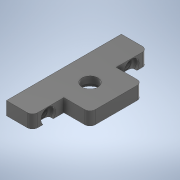
# Autodesk Inventor part: КрепежРадиатора
Saved by Autodesk Inventor 2020 (Build 240168000, 168)
## iProperties
Created: 2020-04-05
Part Number: КрепежРадиатора
Material: Типовые
Document SubType Name: Modeling
Designer: Михаил
Density: 1 g/cm^3
Appearance: По умолчанию
Author: Михаил
Autodesk Inventor part; units mm, degrees
ref_plane "YZ Plane" through (0, 0, 0) normal (1, 0, 0) x (0, 1, 0)
ref_plane "XZ Plane" through (0, 0, 0) normal (0, 1, 0) x (-1, 0, 0)
ref_plane "XY Plane" through (0, 0, 0) normal (0, 0, 1) x (1, 0, 0)
sketch "Эскиз1" plane through (0, 0, 0) normal (0, 1, 0) x (-1, 0, 0)
  line L0 (0, 0) -> (20, 0)
  line L1 (20, 0) -> (20, -20)
  line L2 (20, -20) -> (0, -20)
  line L3 (0, -20) -> (0, 0)
  dimension "d0" = 20
  dimension "d1" = 20
  constraints: 8 end point, 2 parallel, 1 horizontal, 1 perpendicular
  measures "d0" distance of L1.end L2.end
  measures "d1" distance of L0.end L1.end
extrude "Выдавливание1" add sketch "Эскиз1" along normal blind 5
sketch "Эскиз2" plane through (-20, 0, -20) normal (-1, 0, 0) x (0, 0, 1)
  line L0 (0, 5) -> (20, 5) projected
  line L1 (20, 5) -> (32, 5)
  line L2 (32, 5) -> (32, 0)
  line L3 (32, 0) -> (20, 0)
  line L4 (20, 0) -> (20, 5)
  line L5 (0, 0) -> (0, 5) projected
  line L6 (0, 5) -> (-12, 5)
  line L7 (-12, 5) -> (-12, 0)
  line L8 (-12, 0) -> (0, 0)
  line L9 (0, 0) -> (0, 5)
  point P0 (20, 0)
  point P1 (0, 0)
  dimension "d4" = 12
  dimension "d5" = 5
  dimension "d6" = 12
  dimension "d7" = 5
  constraints: 16 end point, 4 parallel, 2 horizontal, 2 perpendicular
  measures "d4" distance of L2.end L3.end
  measures "d5" distance between parallel lines of L1 L3
  measures "d6" distance of L8.end L7.end
  measures "d7" distance between parallel lines of L8 L6
extrude "Выдавливание2" add sketch "Эскиз2" against normal blind 10
sketch "Эскиз4" plane through (-10, 0, -20) normal (1, 0, 0) x (0, 0, -1)
  circle A0 centre (-26, 2) radius 1.55
  circle A1 centre (6, 2) radius 1.55
  line L0 (-32, 5) -> (-32, 0) projected
  line L1 (12, 0) -> (12, 5) projected
  line L2 (-32, 0) -> (-20, 0) projected
  line L3 (0, 0) -> (12, 0) projected
  dimension "d14" = 3.1
  dimension "d15" = 3.1
  dimension "d16" = 6
  dimension "d17" = 6
  dimension "d18" = 2
  dimension "d19" = 2
  constraints: 2 centre point
  measures "d14" diameter of A0
  measures "d15" diameter of A1
  measures "d16" distance from line of L0 A0.centre
  measures "d17" distance from line of L1 A1.centre
  measures "d18" distance from line of L2 A0.centre
  measures "d19" distance from line of L3 A1.centre
sketch "Эскиз5" plane through (-10, 0, -20) normal (1, 0, 0) x (0, 0, -1)
  circle A0 centre (-26, 2) radius 2.8
  circle A1 centre (6, 2) radius 2.8
  line L0 (-32, 5) -> (-32, 0) projected
  line L1 (12, 0) -> (12, 5) projected
  line L2 (-32, 0) -> (-20, 0) projected
  line L3 (0, 0) -> (12, 0) projected
  point P0 (4.0404, 0)
  point P1 (7.9596, 0)
  point P2 (-27.9596, 0)
  point P3 (-24.0404, 0)
  dimension "d20" = 5.6
  dimension "d21" = 5.6
  dimension "d22" = 6
  dimension "d23" = 6
  dimension "d24" = 2
  dimension "d25" = 2
  constraints: 2 centre point
  measures "d20" diameter of A1
  measures "d21" diameter of A0
  measures "d22" distance from line of L0 A0.centre
  measures "d23" distance from line of L1 A1.centre
  measures "d24" distance from line of L2 A0.centre
  measures "d25" distance from line of L3 A1.centre
sketch "Эскиз6" plane through (0, 5, 0) normal (0, 1, 0) x (1, 0, 0)
  circle A0 centre (-10, 10) radius 3.05
  line L0 (-20, -12) -> (-20, 32) projected
  line L1 (-10, 0) -> (0, 0) projected
  dimension "d26" = 6.1
  dimension "d27" = 10
  dimension "d28" = 10
  constraints: 1 centre point
  measures "d26" diameter of A0
  measures "d27" distance from line of L0 A0.centre
  measures "d28" distance from line of L1 A0.centre
sketch "Эскиз7" plane through (0, 0, 0) normal (0, 1, 0) x (1, 0, 0)
  circle A0 centre (-10, 10) radius 5.3
  line L0 (-20, -12) -> (-20, 32) projected
  line L1 (-10, 0) -> (0, 0) projected
  dimension "d29" = 10.6
  dimension "d30" = 10
  dimension "d31" = 10
  constraints: 1 centre point
  measures "d29" diameter of A0
  measures "d30" distance from line of L0 A0.centre
  measures "d31" distance from line of L1 A0.centre
fillet "Сопряжение1" radius 2 4 edges at (0, 2.5, 0) (0, 2.5, -20) (-10, 2.5, 12) (-10, 2.5, -32)
extrude "Выдавливание3" cut sketch "Эскиз4" against normal blind 10
extrude "Выдавливание4" cut sketch "Эскиз6" against normal blind 10
extrude "Выдавливание5" cut sketch "Эскиз5" against normal blind 2 contours A0 L2 | A1 L3 picked at (-25.2881, 1.9538) picked at (6.0159, 2.85)
fillet "Сопряжение2" radius 1 1 edges at (-12, 4.8, 6)
fillet "Сопряжение3" radius 1 1 edges at (-12, 4.8, -26)
extrude "Выдавливание6" cut sketch "Эскиз7" along normal blind 2.4
fillet "Сопряжение4" radius 1 1 edges at (-15.3, 2.4, -10)
